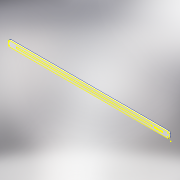
# Autodesk Inventor part: 2021-01-007
Saved by Autodesk Inventor 2020.2 (Build 242310000, 310)
## iProperties
Created: 2020-10-04
Part Number: 2021-01-007
Material: Aluminum 6061
Document SubType Name: Modeling
Designer: carso
Density: 2.7 g/cm^3
Appearance: Aluminum - Flat
Mass: 37.1945 g
Surface Area: 115.588 cm^2
Volume: 13.7758 cm^3
Author: carso
Autodesk Inventor part; units mm, degrees
ref_plane "YZ Plane" through (0, 0, 0) normal (1, 0, 0) x (0, 1, 0)
ref_plane "XZ Plane" through (0, 0, 0) normal (0, 1, 0) x (-1, 0, 0)
ref_plane "XY Plane" through (0, 0, 0) normal (0, 0, 1) x (1, 0, 0)
sketch "Sketch1" plane through (0, 0, 0) normal (0, 0, 1) x (1, 0, 0)
  line L0 (-381.35, 16.05) -> (-6, 16.05)
  line L1 (-3, 13.05) -> (-3, 6)
  line L2 (-6, 3) -> (-381.35, 3)
  line L3 (-384.35, 6) -> (-384.35, 13.05)
  arc A0 (-3, 13.05) -> (-6, 16.05) centre (-6, 13.05) ccw
  arc A1 (-6, 3) -> (-3, 6) centre (-6, 6) ccw
  arc A2 (-381.35, 16.05) -> (-384.35, 13.05) centre (-381.35, 13.05) ccw
  arc A3 (-384.35, 6) -> (-381.35, 3) centre (-381.35, 6) ccw
  line L4 (-41.8897, 11.0236) -> (-317.4797, 11.0236)
  line L5 (-317.4797, 7.9756) -> (-41.8897, 7.9756)
  line L6 (-368.2797, 11.0236) -> (-368.2797, 7.9756)
  arc A4 (-368.2797, 11.0236) -> (-368.2797, 7.9756) centre (-368.2797, 9.4996) ccw
  line L7 (-86.8832, 11.0236) -> (-99.5832, 11.0236)
  line L8 (-41.8897, 11.0236) -> (-41.8897, 7.9756)
  arc A5 (-41.8897, 7.9756) -> (-41.8897, 11.0236) centre (-41.8897, 9.4996) ccw
  line L9 (-36.3424, 11.0744) -> (-6.7422, 11.0744) construction
  line L10 (-6.7422, 11.0744) -> (-6.7422, 8.0311) construction
  line L11 (-6.7422, 8.0311) -> (-36.3424, 8.0311) construction
  line L12 (-36.3424, 8.0311) -> (-36.3424, 11.0744) construction
  line L13 (-317.4797, 11.0236) -> (-368.2797, 11.0236)
  line L14 (-317.4797, 7.9756) -> (-368.2797, 7.9756)
  line L15 (-193.675, 9.525) -> (-193.675, 10.1012)
  line L16 (-193.675, 9.525) -> (-193.6526, 8.8818)
  line L17 (-35.1521, 9.2905) -> (-35.4935, 8.9245)
  line L18 (-35.4935, 8.9245) -> (-35.4935, 7.9833)
  line L19 (-35.4935, 7.9833) -> (-36.0379, 7.9833)
  line L20 (-36.0379, 7.9833) -> (-36.0379, 11.0313)
  line L21 (-36.0379, 11.0313) -> (-35.4935, 11.0313)
  line L22 (-35.4935, 11.0313) -> (-35.4935, 9.6073)
  line L23 (-35.4935, 9.6073) -> (-35.2013, 9.9733)
  line L24 (-35.2013, 9.9733) -> (-34.3278, 11.0313)
  line L25 (-34.3278, 11.0313) -> (-33.6665, 11.0313)
  line L26 (-33.6665, 11.0313) -> (-34.7922, 9.6842)
  line L27 (-34.7922, 9.6842) -> (-33.6081, 7.9833)
  line L28 (-33.6081, 7.9833) -> (-34.254, 7.9833)
  line L29 (-34.254, 7.9833) -> (-35.1521, 9.2905)
  spline S0 degree 2 poles (-31.6581, 9.5704) (-31.4028, 9.5027) (-31.1445, 9.1244) (-31.1445, 8.8753) knots 0 0 0 1 2 2 2
  spline S1 degree 2 poles (-31.1445, 8.8753) (-31.1445, 8.4416) (-31.7012, 7.9833) (-32.2056, 7.9833) knots 0 0 0 1 2 2 2
  line L30 (-32.2056, 7.9833) -> (-33.1252, 7.9833)
  line L31 (-33.1252, 7.9833) -> (-33.3313, 7.9833)
  line L32 (-33.3313, 7.9833) -> (-33.3313, 11.0313)
  line L33 (-33.3313, 11.0313) -> (-32.2825, 11.0313)
  spline S2 degree 2 poles (-32.2825, 11.0313) (-31.7688, 11.0313) (-31.2152, 10.6223) (-31.2152, 10.2071) knots 0 0 0 1 2 2 2
  spline S3 degree 2 poles (-31.2152, 10.2071) (-31.2152, 9.9918) (-31.4428, 9.6596) (-31.6581, 9.5704) knots 0 0 0 1 2 2 2
  spline S4 degree 2 poles (-32.2056, 8.4201) (-31.9534, 8.4201) (-31.6858, 8.6692) (-31.6858, 8.8753) knots 0 0 0 1 2 2 2
  spline S5 degree 2 poles (-31.6858, 8.8753) (-31.6858, 9.352) (-32.184, 9.352) knots 0 0 0 1 1 1
  line L34 (-32.184, 9.352) -> (-32.7869, 9.352)
  line L35 (-32.7869, 9.352) -> (-32.7869, 8.4201)
  line L36 (-32.7869, 8.4201) -> (-32.2056, 8.4201)
  line L37 (-32.7869, 10.5946) -> (-32.7869, 9.7488)
  line L38 (-32.7869, 9.7488) -> (-32.2794, 9.7488)
  spline S6 degree 2 poles (-32.2794, 9.7488) (-32.0303, 9.7488) (-31.7565, 9.9733) (-31.7565, 10.1732) knots 0 0 0 1 2 2 2
  spline S7 degree 2 poles (-31.7565, 10.1732) (-31.7565, 10.3947) (-32.0118, 10.5946) (-32.2825, 10.5946) knots 0 0 0 1 2 2 2
  line L39 (-32.2825, 10.5946) -> (-32.7869, 10.5946)
  spline S8 degree 2 poles (-29.7143, 11.0313) (-29.3083, 11.0313) (-28.6839, 10.6715) (-28.3364, 10.0133) (-28.3364, 9.5796) knots 0 0 0 1 2 3 3 3
  line L40 (-28.3364, 9.5796) -> (-28.3364, 9.432)
  spline S9 degree 2 poles (-28.3364, 9.432) (-28.3364, 8.9952) (-28.6839, 8.3401) (-29.3144, 7.9833) (-29.7327, 7.9833) knots 0 0 0 1 2 3 3 3
  line L41 (-29.7327, 7.9833) -> (-30.3786, 7.9833)
  line L42 (-30.3786, 7.9833) -> (-30.6185, 7.9833)
  line L43 (-30.6185, 7.9833) -> (-30.6185, 11.0313)
  line L44 (-30.6185, 11.0313) -> (-30.0741, 11.0313)
  line L45 (-30.0741, 11.0313) -> (-29.7143, 11.0313)
  spline S10 degree 2 poles (-28.8808, 9.5858) (-28.8808, 10.0748) (-29.3083, 10.5946) (-29.7143, 10.5946) knots 0 0 0 1 2 2 2
  line L46 (-29.7143, 10.5946) -> (-30.0741, 10.5946)
  line L47 (-30.0741, 10.5946) -> (-30.0741, 8.4201)
  line L48 (-30.0741, 8.4201) -> (-29.7327, 8.4201)
  spline S11 degree 2 poles (-29.7327, 8.4201) (-29.3144, 8.4201) (-28.8808, 8.9491) (-28.8808, 9.432) knots 0 0 0 1 2 2 2
  line L49 (-28.8808, 9.432) -> (-28.8808, 9.5858)
  line L50 (-26.8293, 7.9833) -> (-26.8293, 8.3432)
  line L51 (-26.8293, 8.3432) -> (-25.8389, 9.4197)
  spline S12 degree 2 poles (-25.8389, 9.4197) (-25.6759, 9.6011) (-25.4914, 9.8626) (-25.4145, 10.0717) (-25.4145, 10.1763) knots 0 0 0 1 2 3 3 3
  spline S13 degree 2 poles (-25.4145, 10.1763) (-25.4145, 10.3916) (-25.6513, 10.6561) (-25.8604, 10.6561) knots 0 0 0 1 2 2 2
  spline S14 degree 2 poles (-25.8604, 10.6561) (-26.1065, 10.6561) (-26.3679, 10.3516) (-26.3679, 10.0994) knots 0 0 0 1 2 2 2
  line L52 (-26.3679, 10.0994) -> (-26.8908, 10.0994)
  spline S15 degree 2 poles (-26.8908, 10.0994) (-26.8908, 10.3701) (-26.6417, 10.813) (-26.1742, 11.0744) (-25.8543, 11.0744) knots 0 0 0 1 2 3 3 3
  spline S16 degree 2 poles (-25.8543, 11.0744) (-25.5498, 11.0744) (-25.1192, 10.8683) (-24.8916, 10.49) (-24.8916, 10.2317) knots 0 0 0 1 2 3 3 3
  spline S17 degree 2 poles (-24.8916, 10.2317) (-24.8916, 9.9641) (-25.2115, 9.4289) (-25.516, 9.109) knots 0 0 0 1 2 2 2
  line L53 (-25.516, 9.109) -> (-26.1772, 8.4016)
  line L54 (-26.1772, 8.4016) -> (-24.7747, 8.4016)
  line L55 (-24.7747, 8.4016) -> (-24.7747, 7.9833)
  line L56 (-24.7747, 7.9833) -> (-26.8293, 7.9833)
  spline S18 degree 2 poles (-23.2184, 10.0071) (-22.9324, 10.0071) (-22.5387, 9.7242) (-22.348, 9.2597) (-22.348, 8.9829) knots 0 0 0 1 2 3 3 3
  spline S19 degree 2 poles (-22.348, 8.9829) (-22.348, 8.6877) (-22.5848, 8.214) (-23.037, 7.9403) (-23.3415, 7.9403) knots 0 0 0 1 2 3 3 3
  spline S20 degree 2 poles (-23.3415, 7.9403) (-23.6613, 7.9403) (-24.1288, 8.2663) (-24.3749, 8.8138) (-24.3749, 9.1398) knots 0 0 0 1 2 3 3 3
  line L57 (-24.3749, 9.1398) -> (-24.3749, 9.3428)
  spline S21 degree 2 poles (-24.3749, 9.3428) (-24.3749, 9.8226) (-24.0612, 10.5915) (-23.3814, 11.0498) (-22.8617, 11.0498) knots 0 0 0 1 2 3 3 3
  line L58 (-22.8617, 11.0498) -> (-22.7971, 11.0498)
  line L59 (-22.7971, 11.0498) -> (-22.7971, 10.6192)
  line L60 (-22.7971, 10.6192) -> (-22.834, 10.6192)
  spline S22 degree 2 poles (-22.834, 10.6192) (-23.1477, 10.6192) (-23.5783, 10.3916) (-23.812, 10.0071) (-23.8397, 9.7519) knots 0 0 0 1 2 3 3 3
  spline S23 degree 2 poles (-23.8397, 9.7519) (-23.7259, 9.8749) (-23.4061, 10.0071) (-23.2184, 10.0071) knots 0 0 0 1 2 2 2
  spline S24 degree 2 poles (-23.3476, 8.3616) (-23.2, 8.3616) (-22.9816, 8.5185) (-22.8647, 8.7922) (-22.8647, 8.9706) knots 0 0 0 1 2 3 3 3
  spline S25 degree 2 poles (-22.8647, 8.9706) (-22.8647, 9.1429) (-22.9785, 9.4228) (-23.1969, 9.5858) (-23.3507, 9.5858) knots 0 0 0 1 2 3 3 3
  spline S26 degree 2 poles (-23.3507, 9.5858) (-23.5199, 9.5858) (-23.7905, 9.3951) (-23.852, 9.2505) knots 0 0 0 1 2 2 2
  line L61 (-23.852, 9.2505) -> (-23.852, 9.0906)
  spline S27 degree 2 poles (-23.852, 9.0906) (-23.852, 8.8599) (-23.7167, 8.5308) (-23.4891, 8.3616) (-23.3476, 8.3616) knots 0 0 0 1 2 3 3 3
  spline S28 degree 2 poles (-19.9521, 9.2659) (-19.9521, 7.9403) (-20.9486, 7.9403) knots 0 0 0 1 1 1
  spline S29 degree 2 poles (-20.9486, 7.9403) (-21.4253, 7.9403) (-21.9543, 8.5739) (-21.9543, 9.2659) knots 0 0 0 1 2 2 2
  line L62 (-21.9543, 9.2659) -> (-21.9543, 9.7642)
  spline S30 degree 2 poles (-21.9543, 9.7642) (-21.9543, 10.4531) (-21.4315, 11.0744) (-20.9547, 11.0744) knots 0 0 0 1 2 2 2
  spline S31 degree 2 poles (-20.9547, 11.0744) (-20.478, 11.0744) (-19.9521, 10.4531) (-19.9521, 9.7642) knots 0 0 0 1 2 2 2
  line L63 (-19.9521, 9.7642) -> (-19.9521, 9.2659)
  spline S32 degree 2 poles (-20.4719, 9.8411) (-20.4719, 10.2809) (-20.7118, 10.6561) (-20.9547, 10.6561) knots 0 0 0 1 2 2 2
  spline S33 degree 2 poles (-20.9547, 10.6561) (-21.1916, 10.6561) (-21.4345, 10.2809) (-21.4345, 9.8411) knots 0 0 0 1 2 2 2
  line L64 (-21.4345, 9.8411) -> (-21.4345, 9.1921)
  spline S34 degree 2 poles (-21.4345, 9.1921) (-21.4345, 8.7523) (-21.1885, 8.3616) (-20.9486, 8.3616) knots 0 0 0 1 2 2 2
  spline S35 degree 2 poles (-20.9486, 8.3616) (-20.7087, 8.3616) (-20.4719, 8.7461) (-20.4719, 9.1921) knots 0 0 0 1 2 2 2
  line L65 (-20.4719, 9.1921) -> (-20.4719, 9.8411)
  spline S36 degree 2 poles (-17.51, 9.2659) (-17.51, 7.9403) (-18.5065, 7.9403) knots 0 0 0 1 1 1
  spline S37 degree 2 poles (-18.5065, 7.9403) (-18.9832, 7.9403) (-19.5122, 8.5739) (-19.5122, 9.2659) knots 0 0 0 1 2 2 2
  line L66 (-19.5122, 9.2659) -> (-19.5122, 9.7642)
  spline S38 degree 2 poles (-19.5122, 9.7642) (-19.5122, 10.4531) (-18.9894, 11.0744) (-18.5126, 11.0744) knots 0 0 0 1 2 2 2
  spline S39 degree 2 poles (-18.5126, 11.0744) (-18.0359, 11.0744) (-17.51, 10.4531) (-17.51, 9.7642) knots 0 0 0 1 2 2 2
  line L67 (-17.51, 9.7642) -> (-17.51, 9.2659)
  spline S40 degree 2 poles (-18.0298, 9.8411) (-18.0298, 10.2809) (-18.2697, 10.6561) (-18.5126, 10.6561) knots 0 0 0 1 2 2 2
  spline S41 degree 2 poles (-18.5126, 10.6561) (-18.7495, 10.6561) (-18.9925, 10.2809) (-18.9925, 9.8411) knots 0 0 0 1 2 2 2
  line L68 (-18.9925, 9.8411) -> (-18.9925, 9.1921)
  spline S42 degree 2 poles (-18.9925, 9.1921) (-18.9925, 8.7523) (-18.7464, 8.3616) (-18.5065, 8.3616) knots 0 0 0 1 2 2 2
  spline S43 degree 2 poles (-18.5065, 8.3616) (-18.2666, 8.3616) (-18.0298, 8.7461) (-18.0298, 9.1921) knots 0 0 0 1 2 2 2
  line L69 (-18.0298, 9.1921) -> (-18.0298, 9.8411)
  point P0 (0, 0)
  point P1 (0, 0)
  point P2 (0, 0)
  point P3 (-31.75, 11.049)
  point P4 (-31.75, 8.001)
  point P5 (19.05, 8.001)
  point P6 (19.05, 11.049)
  dimension "d0" = 3
  constraints: 26 end point, 12 point on circle, 9 tangent, 6 centre point, 3 equal radius, 3 horizontal, 2 parallel, 1 perpendicular, 1 vertical, 2 other
  measures "d0" radius of A0
extrude "Extrusion1" add sketch "Sketch1" against normal blind 3 contours L0 A0 L1 A1 L2 A3 L3 A2 | L8 L5 L14 L6 L13 L4 | A5 L8 | A4 L6 | L17 L18 L19 L20 L21 L22 L23 L24 L25 L26 L27 L28 L29 | S0 S1 L30 L31 L32 L33 S2 S3 | L36 L35 L34 S5 S4 | L39 S7 S6 L38 L37 | S8 L40 S9 L41 L42 L43 L44 L45 | L49 S11 L48 L47 L46 S10 | L50 L51 S12 S13 S14 L52 S15 S16 S17 L53 L54 L55 L56 | S18 S19 S20 L57 S21 L58 L59 L60 S22 S23 | S27 L61 S26 S25 S24 | S28 S29 L62 S30 S31 L63 | L65 S35 S34 L64 S33 S32 | S36 S37 L66 S38 S39 L67 | L69 S43 S42 L68 S41 S40
extrude "Extrusion2" cut sketch "Sketch1" against normal blind 0.1 contours L8 L5 L14 L6 L13 L4 | A5 L8 | A4 L6 | L17 L18 L19 L20 L21 L22 L23 L24 L25 L26 L27 L28 L29 | S0 S1 L30 L31 L32 L33 S2 S3 | S8 L40 S9 L41 L42 L43 L44 L45 | L50 L51 S12 S13 S14 L52 S15 S16 S17 L53 L54 L55 L56 | S18 S19 S20 L57 S21 L58 L59 L60 S22 S23 | S28 S29 L62 S30 S31 L63 | S36 S37 L66 S38 S39 L67
sketch "Sketch2" plane through (0, 0, 0) normal (0, 0, 1) x (1, 0, 0)
  line L0 (-6, 16.05) -> (-381.35, 16.05) projected
  line L1 (-3, 3) -> (-355.95, 3)
  line L2 (-358.95, 6) -> (-358.95, 13.05)
  line L3 (-355.95, 16.05) -> (-3, 16.05)
  line L4 (-3, 16.05) -> (-3, 3)
  arc A0 (-355.95, 16.05) -> (-358.95, 13.05) centre (-355.95, 13.05) ccw
  arc A1 (-358.95, 6) -> (-355.95, 3) centre (-355.95, 6) ccw
  line L5 (-355.95, 16.05) -> (-339.88, 16.05)
  line L6 (-339.88, 7.9756) -> (-355.95, 7.9756)
  arc A2 (-339.88, 11.0236) -> (-339.88, 7.9756) centre (-339.88, 9.4996) ccw
  line L7 (-358.95, 11.0236) -> (-339.88, 11.0236)
  line L8 (-339.88, 11.0236) -> (-339.88, 7.9756)
  line L9 (-339.88, 7.9756) -> (-358.95, 7.9756)
  line L10 (-358.95, 7.9756) -> (-358.95, 11.0236)
  line L11 (-355.95, 16.05) -> (-390.1451, 16.05)
  line L12 (-390.1451, 16.05) -> (-390.1451, 0)
  line L13 (-390.1451, 0) -> (-355.95, 0)
  line L14 (-355.95, 0) -> (-355.95, 3)
  point P0 (0, 0)
  point P1 (-358.95, 16.05)
  constraints: 28 end point, 6 point on circle, 5 parallel, 5 perpendicular, 5 tangent, 4 horizontal, 4 point on line, 3 centre point, 1 equal radius
extrude "Extrusion3" cut sketch "Sketch2" against normal blind 10 contours A0 L2 A1 L14 L13 L12 L11 L0
extrude "Extrusion4" add sketch "Sketch2" against normal up to surface (0.1 mm away) contours L7 A2 L6 L9 L2
sketch "Sketch3" plane through (0, 0, -3) normal (0, 0, -1) x (-1, 0, 0)
  line L0 (3, 16.05) -> (358.95, 16.05)
  line L1 (358.95, 16.05) -> (358.95, 3)
  line L2 (358.95, 3) -> (3, 3)
  line L3 (3, 3) -> (3, 16.05)
  line L4 (355.95, 3) -> (6, 3) projected
  line L5 (3, 16.05) -> (33, 16.05)
  line L6 (33, 16.05) -> (33, 3)
  line L7 (33, 3) -> (3, 3)
  line L8 (3, 3) -> (3, 16.05)
  line L9 (358.95, 16.05) -> (328.95, 16.05)
  line L10 (328.95, 16.05) -> (328.95, 3)
  line L11 (328.95, 3) -> (358.95, 3)
  line L12 (358.95, 3) -> (358.95, 16.05)
  line L13 (33, 16.05) -> (33, 9.525)
  line L14 (33, 9.525) -> (328.95, 9.525)
  line L15 (33, 9.525) -> (63, 9.525)
  line L16 (328.95, 9.525) -> (298.95, 9.525)
  circle A0 centre (63, 9.525) radius 2.5
  circle A1 centre (298.95, 9.525) radius 2.5
  line L17 (65.5, 9.525) -> (70.5, 9.525)
  point P0 (0, 0)
  dimension "d20" = 30
  dimension "d21" = 30
  dimension "d22" = 6.525
  dimension "d23" = 30
  dimension "d24" = 30
  dimension "d26" = 5
  dimension "d27" = 5
  constraints: 34 end point, 6 parallel, 6 point on line, 3 horizontal, 3 perpendicular, 2 coincident, 2 midpoint, 1 centre point, 1 horizontal alignment, 2 other
  measures "d20" distance of L6.end L7.end
  measures "d21" distance of L11.end L10.end
  measures "d22" distance of L5.end L13.end
  measures "d23" distance of L13.end L15.end
  measures "d24" distance of L14.end L16.end
  measures "d26" diameter of A1
  measures "d27" distance of L17.start L17.end
extrude "Extrusion5" cut sketch "Sketch3" against normal blind 1 contours A0 L14 | L14 A0 | A1 L14 | L14 A1
sketch "Sketch4" plane through (-298.95, 9.525, -2) normal (0, 0, -1) x (-1, 0, 0)
  circle A0 centre (-235.95, 0) radius 2.5 projected
  circle A1 centre (-235.95, 0) radius 2.5
  circle A2 centre (-235.95, 0) radius 1.5
  circle A3 centre (0, 0) radius 2.5
  circle A4 centre (0, 0) radius 1.5
  point P0 (-298.95, -9.525)
  dimension "d30" = 1
  dimension "d31" = 1
  constraints: 4 centre point, 1 coincident
  measures "d30" radial gap between concentric circles of A0 A2
  measures "d31" radial gap between concentric circles of A3 A4
extrude "Extrusion6" cut sketch "Sketch4" against normal blind 0.2 contours A2 | A4
sketch "Sketch5" plane through (0, 0, 0) normal (0, 0, 1) x (1, 0, 0)
  line L0 (-358.95, 13.05) -> (-358.95, 6) projected
  arc A0 (-358.95, 6) -> (-355.95, 3) centre (-355.95, 6) ccw projected
  line L1 (-355.95, 3) -> (-6, 3) projected
  arc A1 (-6, 3) -> (-3, 6) centre (-6, 6) ccw projected
  line L2 (-3, 6) -> (-3, 13.05) projected
  arc A2 (-3, 13.05) -> (-6, 16.05) centre (-6, 13.05) ccw projected
  line L3 (-6, 16.05) -> (-355.95, 16.05) projected
  arc A3 (-355.95, 16.05) -> (-358.95, 13.05) centre (-355.95, 13.05) ccw projected
  line L4 (-355.95, 16.075) -> (-6, 16.075)
  arc A4 (-2.975, 13.05) -> (-6, 16.075) centre (-6, 13.05) ccw
  line L5 (-2.975, 13.05) -> (-2.975, 6)
  arc A5 (-6, 2.975) -> (-2.975, 6) centre (-6, 6) ccw
  line L6 (-6, 2.975) -> (-355.95, 2.975)
  arc A6 (-358.975, 6) -> (-355.95, 2.975) centre (-355.95, 6) ccw
  line L7 (-358.975, 6) -> (-358.975, 13.05)
  arc A7 (-355.95, 16.075) -> (-358.975, 13.05) centre (-355.95, 13.05) ccw
  point P0 (0, 0)
  dimension "d34" = 0.025
  constraints: 8 end point, 8 point on circle, 4 centre point, 7 other
  measures "d34" distance between parallel lines of L3 L4
extrude "Extrusion7" add sketch "Sketch5" against normal up to surface (3 mm away)
sketch "Sketch6" plane through (0, 0, 0) normal (0, 0, 1) x (1, 0, 0)
  arc A0 (-6, 2.975) -> (-2.975, 6) centre (-6, 6) ccw projected
  line L0 (-2.975, 6) -> (-2.975, 13.05) projected
  arc A1 (-2.975, 13.05) -> (-6, 16.075) centre (-6, 13.05) ccw projected
  line L1 (-6, 16.075) -> (-355.95, 16.075) projected
  arc A2 (-355.95, 16.075) -> (-358.975, 13.05) centre (-355.95, 13.05) ccw projected
  line L2 (-358.975, 13.05) -> (-358.975, 6) projected
  arc A3 (-358.975, 6) -> (-355.95, 2.975) centre (-355.95, 6) ccw projected
  line L3 (-355.95, 2.975) -> (-6, 2.975) projected
  line L4 (-355.95, 15.875) -> (-6, 15.875)
  arc A4 (-3.175, 13.05) -> (-6, 15.875) centre (-6, 13.05) ccw
  line L5 (-3.175, 13.05) -> (-3.175, 6)
  arc A5 (-6, 3.175) -> (-3.175, 6) centre (-6, 6) ccw
  line L6 (-6, 3.175) -> (-355.95, 3.175)
  arc A6 (-358.775, 6) -> (-355.95, 3.175) centre (-355.95, 6) ccw
  line L7 (-358.775, 6) -> (-358.775, 13.05)
  arc A7 (-355.95, 15.875) -> (-358.775, 13.05) centre (-355.95, 13.05) ccw
  point P0 (0, 0)
  dimension "d37" = 0.2
  constraints: 8 end point, 8 point on circle, 4 centre point, 7 other
  measures "d37" distance between parallel lines of L1 L4
extrude "Extrusion8" cut sketch "Sketch6" against normal blind 10
sketch "Sketch7" plane through (0, 0, 0) normal (0, 0, 1) x (1, 0, 0)
  line L0 (-18.0298, 9.1921) -> (-18.0298, 9.8411) projected
  line L1 (-18.9925, 9.8411) -> (-18.9925, 9.1921) projected
  line L2 (-17.51, 9.7642) -> (-17.51, 9.2659) projected
  line L3 (-19.5122, 9.2659) -> (-19.5122, 9.7642) projected
  line L4 (-20.4719, 9.1921) -> (-20.4719, 9.8411) projected
  line L5 (-21.4345, 9.8411) -> (-21.4345, 9.1921) projected
  line L6 (-19.9521, 9.7642) -> (-19.9521, 9.2659) projected
  line L7 (-21.9543, 9.2659) -> (-21.9543, 9.7642) projected
  line L8 (-23.852, 9.2505) -> (-23.852, 9.0906) projected
  line L9 (-22.7971, 10.6192) -> (-22.834, 10.6192) projected
  line L10 (-22.7971, 11.0498) -> (-22.7971, 10.6192) projected
  line L11 (-22.8617, 11.0498) -> (-22.7971, 11.0498) projected
  line L12 (-24.3749, 9.1398) -> (-24.3749, 9.3428) projected
  line L13 (-26.8293, 7.9833) -> (-26.8293, 8.3432) projected
  line L14 (-24.7747, 7.9833) -> (-26.8293, 7.9833) projected
  line L15 (-24.7747, 8.4016) -> (-24.7747, 7.9833) projected
  line L16 (-26.1772, 8.4016) -> (-24.7747, 8.4016) projected
  line L17 (-25.516, 9.109) -> (-26.1772, 8.4016) projected
  line L18 (-26.3679, 10.0994) -> (-26.8908, 10.0994) projected
  line L19 (-26.8293, 8.3432) -> (-25.8389, 9.4197) projected
  line L20 (-29.7143, 10.5946) -> (-30.0741, 10.5946) projected
  line L21 (-28.8808, 9.432) -> (-28.8808, 9.5858) projected
  line L22 (-30.0741, 8.4201) -> (-29.7327, 8.4201) projected
  line L23 (-30.0741, 10.5946) -> (-30.0741, 8.4201) projected
  line L24 (-30.6185, 11.0313) -> (-29.7143, 11.0313) projected
  line L25 (-30.6185, 7.9833) -> (-30.6185, 11.0313) projected
  line L26 (-29.7327, 7.9833) -> (-30.6185, 7.9833) projected
  line L27 (-28.3364, 9.5796) -> (-28.3364, 9.432) projected
  line L28 (-32.7869, 9.7488) -> (-32.2794, 9.7488) projected
  line L29 (-32.7869, 10.5946) -> (-32.7869, 9.7488) projected
  line L30 (-32.2825, 10.5946) -> (-32.7869, 10.5946) projected
  line L31 (-32.7869, 8.4201) -> (-32.2056, 8.4201) projected
  line L32 (-32.7869, 9.352) -> (-32.7869, 8.4201) projected
  line L33 (-32.184, 9.352) -> (-32.7869, 9.352) projected
  line L34 (-33.3313, 11.0313) -> (-32.2825, 11.0313) projected
  line L35 (-33.3313, 7.9833) -> (-33.3313, 11.0313) projected
  line L36 (-32.2056, 7.9833) -> (-33.3313, 7.9833) projected
  line L37 (-35.1521, 9.2905) -> (-35.4935, 8.9245) projected
  line L38 (-34.254, 7.9833) -> (-35.1521, 9.2905) projected
  line L39 (-33.6081, 7.9833) -> (-34.254, 7.9833) projected
  line L40 (-34.7922, 9.6842) -> (-33.6081, 7.9833) projected
  line L41 (-33.6665, 11.0313) -> (-34.7922, 9.6842) projected
  line L42 (-34.3278, 11.0313) -> (-33.6665, 11.0313) projected
  line L43 (-35.2013, 9.9733) -> (-34.3278, 11.0313) projected
  line L44 (-35.4935, 9.6073) -> (-35.2013, 9.9733) projected
  line L45 (-35.4935, 11.0313) -> (-35.4935, 9.6073) projected
  line L46 (-36.0379, 11.0313) -> (-35.4935, 11.0313) projected
  line L47 (-36.0379, 7.9833) -> (-36.0379, 11.0313) projected
  line L48 (-35.4935, 7.9833) -> (-36.0379, 7.9833) projected
  line L49 (-35.4935, 8.9245) -> (-35.4935, 7.9833) projected
  arc A0 (-339.88, 11.0236) -> (-339.88, 7.9756) centre (-339.88, 9.4996) ccw projected
  line L50 (-41.8897, 7.9756) -> (-339.88, 7.9756) projected
  arc A1 (-41.8897, 7.9756) -> (-41.8897, 11.0236) centre (-41.8897, 9.4996) ccw projected
  line L51 (-339.88, 11.0236) -> (-41.8897, 11.0236) projected
  arc A2 (-358.775, 6) -> (-355.95, 3.175) centre (-355.95, 6) ccw projected
  line L52 (-355.95, 3.175) -> (-6, 3.175) projected
  arc A3 (-6, 3.175) -> (-3.175, 6) centre (-6, 6) ccw projected
  line L53 (-3.175, 6) -> (-3.175, 13.05) projected
  arc A4 (-3.175, 13.05) -> (-6, 15.875) centre (-6, 13.05) ccw projected
  line L54 (-6, 15.875) -> (-355.95, 15.875) projected
  arc A5 (-355.95, 15.875) -> (-358.775, 13.05) centre (-355.95, 13.05) ccw projected
  line L55 (-358.775, 13.05) -> (-358.775, 6) projected
  line L56 (-24.7747, 7.9833) -> (-26.8293, 7.9833) projected
  line L57 (-26.8293, 7.9833) -> (-26.8293, 8.3432) projected
  line L58 (-26.8293, 8.3432) -> (-25.8389, 9.4197) projected
  line L59 (-26.3679, 10.0994) -> (-26.8908, 10.0994) projected
  line L60 (-25.516, 9.109) -> (-26.1772, 8.4016) projected
  line L61 (-26.1772, 8.4016) -> (-24.7747, 8.4016) projected
  line L62 (-24.7747, 8.4016) -> (-24.7747, 7.9833) projected
  line L63 (-30.6185, 11.0313) -> (-29.7143, 11.0313) projected
  line L64 (-28.3364, 9.5796) -> (-28.3364, 9.432) projected
  line L65 (-29.7327, 7.9833) -> (-30.6185, 7.9833) projected
  line L66 (-30.6185, 7.9833) -> (-30.6185, 11.0313) projected
  line L67 (-34.254, 7.9833) -> (-35.1521, 9.2905) projected
  line L68 (-35.1521, 9.2905) -> (-35.4935, 8.9245) projected
  line L69 (-35.4935, 8.9245) -> (-35.4935, 7.9833) projected
  line L70 (-35.4935, 7.9833) -> (-36.0379, 7.9833) projected
  line L71 (-36.0379, 7.9833) -> (-36.0379, 11.0313) projected
  line L72 (-36.0379, 11.0313) -> (-35.4935, 11.0313) projected
  line L73 (-35.4935, 11.0313) -> (-35.4935, 9.6073) projected
  line L74 (-35.4935, 9.6073) -> (-35.2013, 9.9733) projected
  line L75 (-35.2013, 9.9733) -> (-34.3278, 11.0313) projected
  line L76 (-34.3278, 11.0313) -> (-33.6665, 11.0313) projected
  line L77 (-33.6665, 11.0313) -> (-34.7922, 9.6842) projected
  line L78 (-34.7922, 9.6842) -> (-33.6081, 7.9833) projected
  line L79 (-33.6081, 7.9833) -> (-34.254, 7.9833) projected
  arc A6 (-339.88, 11.0236) -> (-339.88, 7.9756) centre (-339.88, 9.4996) ccw projected
  line L80 (-339.88, 11.0236) -> (-41.8897, 11.0236) projected
  arc A7 (-41.8897, 7.9756) -> (-41.8897, 11.0236) centre (-41.8897, 9.4996) ccw projected
  line L81 (-41.8897, 7.9756) -> (-339.88, 7.9756) projected
  line L82 (-32.2056, 7.9833) -> (-33.3313, 7.9833) projected
  line L83 (-33.3313, 7.9833) -> (-33.3313, 11.0313) projected
  line L84 (-33.3313, 11.0313) -> (-32.2825, 11.0313) projected
  line L85 (-24.3749, 9.1398) -> (-24.3749, 9.3428) projected
  line L86 (-22.8617, 11.0498) -> (-22.7971, 11.0498) projected
  line L87 (-22.7971, 11.0498) -> (-22.7971, 10.6192) projected
  line L88 (-22.7971, 10.6192) -> (-22.834, 10.6192) projected
  line L89 (-19.9521, 9.7642) -> (-19.9521, 9.2659) projected
  line L90 (-21.9543, 9.2659) -> (-21.9543, 9.7642) projected
  line L91 (-17.51, 9.7642) -> (-17.51, 9.2659) projected
  line L92 (-19.5122, 9.2659) -> (-19.5122, 9.7642) projected
  point P0 (0, 0)
  point P1 (-18.5126, 10.6561)
  point P2 (-18.5065, 8.3616)
  point P3 (-18.5065, 7.9403)
  point P4 (-18.5126, 11.0744)
  point P5 (-20.9547, 10.6561)
  point P6 (-20.9486, 8.3616)
  point P7 (-20.9486, 7.9403)
  point P8 (-20.9547, 11.0744)
  point P9 (-23.3507, 9.5858)
  point P10 (-22.8647, 8.9706)
  point P11 (-23.3476, 8.3616)
  point P12 (-22.348, 8.9829)
  point P13 (-23.2184, 10.0071)
  point P14 (-23.8397, 9.7519)
  point P15 (-23.3415, 7.9403)
  point P16 (-24.8916, 10.2317)
  point P17 (-25.8543, 11.0744)
  point P18 (-25.8604, 10.6561)
  point P19 (-25.4145, 10.1763)
  point P20 (-31.7565, 10.1732)
  point P21 (-31.6858, 8.8753)
  point P22 (-31.1445, 8.8753)
  point P23 (-31.6581, 9.5704)
  point P24 (-31.2152, 10.2071)
  point P25 (-25.4145, 10.1763)
  point P26 (-25.8604, 10.6561)
  point P27 (-25.8543, 11.0744)
  point P28 (-24.8916, 10.2317)
  point P29 (-31.2152, 10.2071)
  point P30 (-31.6581, 9.5704)
  point P31 (-31.1445, 8.8753)
  point P32 (-23.8397, 9.7519)
  point P33 (-23.2184, 10.0071)
  point P34 (-22.348, 8.9829)
  point P35 (-23.3415, 7.9403)
  point P36 (-20.9486, 7.9403)
  point P37 (-20.9547, 11.0744)
  point P38 (-18.5065, 7.9403)
  point P39 (-18.5126, 11.0744)
  constraints: 70 other
sketch "Sketch8" plane through (0, 0, 0) normal (0, 0, 1) x (1, 0, 0)
  line L0 (-16.4625, 13.2195) -> (-343.5634, 13.2195)
  line L1 (-343.5634, 13.2195) -> (-343.5634, 5.8328)
  line L2 (-343.5634, 5.8328) -> (-16.4625, 5.8328)
  line L3 (-16.4625, 5.8328) -> (-16.4625, 13.2195)
  point P0 (0, 0)
  constraints: 8 end point, 2 parallel, 1 horizontal, 1 perpendicular
extrude "Extrusion9" add sketch "Sketch8" against normal up to surface (0.1 mm away)
sketch "Sketch9" plane through (0, 0, -3) normal (0, 0, -1) x (-1, 0, 0)
  circle A0 centre (63, 9.525) radius 1.5 projected
  circle A1 centre (63, 9.525) radius 2.55
  circle A2 centre (298.95, 9.525) radius 2.5 projected
  circle A3 centre (298.95, 9.525) radius 2.55
  point P0 (0, 0)
  dimension "d42" = 5.1
  dimension "d43" = 5.1
  constraints: 2 centre point, 2 coincident
  measures "d42" diameter of A1
  measures "d43" diameter of A3
extrude "Extrusion10" cut sketch "Sketch9" against normal up to surface (1 mm away) contours A1 | A2
body "Solid1"
